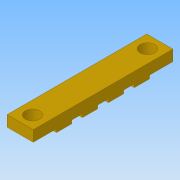
# Autodesk Inventor part: ContactPress
Saved by Autodesk Inventor 2017.3 (Build 213256000, 256)
## iProperties
Created: 2019-06-22
Part Number: ContactPress
Material: ABS Plastic
Document SubType Name: Modeling
Designer: Derek Wider
Density: 1.06 g/cm^3
Appearance: Gold
Author: Derek Wider
Autodesk Inventor part; units mm, degrees
ref_plane "YZ Plane" through (0, 0, 0) normal (1, 0, 0) x (0, 1, 0)
ref_plane "XZ Plane" through (0, 0, 0) normal (0, 1, 0) x (-1, 0, 0)
ref_plane "XY Plane" through (0, 0, 0) normal (0, 0, 1) x (1, 0, 0)
sketch "Sketch1" plane through (0, 0, 0) normal (0, 1, 0) x (-1, 0, 0)
  line L0 (0, 0) -> (6.096, 0)
  line L1 (6.096, 0) -> (6.096, -32.6136)
  line L2 (6.096, -32.6136) -> (0, -32.6136)
  line L3 (0, -32.6136) -> (0, 0)
  dimension "d0" = 6.096
  dimension "d1" = 32.6136
  constraints: 8 end point, 2 parallel, 1 horizontal, 1 perpendicular
  measures "d0" distance of L1.end L2.end
  measures "d1" distance of L0.end L1.end
extrude "Extrusion1" add sketch "Sketch1" along normal blind 2.54
sketch "Sketch2" plane through (0, 0, 0) normal (0, -1, 0) x (1, 0, 0)
  line L0 (0, 0) -> (0, -32.6136) projected
  line L1 (0, -5.4419) -> (-6.096, -5.4419)
  line L2 (-6.096, -5.4419) -> (-6.096, -8.9979)
  line L3 (-6.096, -8.9979) -> (0, -8.9979)
  line L4 (0, -8.9979) -> (0, -5.4419)
  line L5 (0, -11.4998) -> (-6.096, -11.4998)
  line L6 (-6.096, -11.4998) -> (-6.096, -15.0558)
  line L7 (-6.096, -15.0558) -> (0, -15.0558)
  line L8 (0, -15.0558) -> (0, -11.4998)
  line L9 (0, -17.5578) -> (-6.096, -17.5578)
  line L10 (-6.096, -17.5578) -> (-6.096, -21.1138)
  line L11 (-6.096, -21.1138) -> (0, -21.1138)
  line L12 (0, -21.1138) -> (0, -17.5578)
  line L13 (0, -23.6157) -> (-6.096, -23.6157)
  line L14 (-6.096, -23.6157) -> (-6.096, -27.1717)
  line L15 (-6.096, -27.1717) -> (0, -27.1717)
  line L16 (0, -27.1717) -> (0, -23.6157)
  line L17 (-3.048, -8.9979) -> (-3.048, -11.4998) construction
  line L18 (-3.048, -15.0558) -> (-3.048, -17.5578) construction
  line L19 (-3.048, -21.1138) -> (-3.048, -23.6157) construction
  line L20 (-6.096, 0) -> (-6.096, -32.6136) construction
  line L21 (-6.096, 0) -> (0, 0) construction
  line L22 (0, -5.4419) -> (0, 0) construction
  line L23 (0, -32.6136) -> (0, -27.1717) construction
  dimension "d4" = 3.556
  constraints: 42 end point, 8 parallel, 7 collinear, 6 midpoint, 6 point on line, 5 perpendicular, 4 horizontal, 3 vertical alignment
  measures "d4" distance between parallel lines of L1 L3
extrude "Extrusion2" add sketch "Sketch2" along normal blind 0.762
sketch "Sketch3" plane through (0, 0, 0) normal (0, -1, 0) x (1, 0, 0)
  line L0 (0, -5.4419) -> (-6.096, -5.4419) construction
  line L1 (-6.096, -5.4419) -> (-6.096, -8.9979) construction
  line L2 (-6.096, -8.9979) -> (0, -8.9979) construction
  line L3 (0, -8.9979) -> (0, -5.4419) construction
  line L4 (0, -23.6157) -> (-6.096, -23.6157) construction
  line L5 (-6.096, -23.6157) -> (-6.096, -27.1717) construction
  line L6 (-6.096, -27.1717) -> (0, -27.1717) construction
  line L7 (0, -27.1717) -> (0, -23.6157) construction
  circle A0 centre (-3.048, -2.9019) radius 1.7145
  circle A1 centre (-3.048, -29.7117) radius 1.7145
  line L8 (0, -5.4419) -> (-6.096, -5.4419) projected
  line L9 (-6.096, -27.1717) -> (0, -27.1717) projected
  point P0 (0, 0)
  point P1 (-3.048, -5.4419)
  point P2 (-3.048, -27.1717)
  dimension "d7" = 2.54
  dimension "d8" = 2.54
  dimension "d9" = 3.429
  dimension "d10" = 3.429
  constraints: 2 centre point, 2 midpoint, 2 vertical alignment
  measures "d7" distance from line of L0 A0.centre
  measures "d8" distance from line of L6 A1.centre
  measures "d9" diameter of A0
  measures "d10" diameter of A1
extrude "Extrusion3" cut sketch "Sketch3" against normal through all
equation "\"d8\" = d7"
equation "\"d10\" = d9"
body "Solid1"
